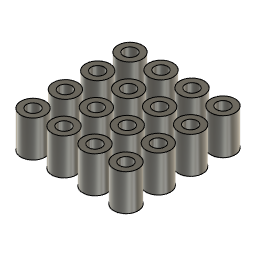
Tall washers v1 (Autodesk Fusion 360 design; units mm, degrees)
Autodesk Fusion 360 part; units mm, degrees
sketch "Sketch1" plane through (0, 0, 0) normal (0, 0, 1) x (1, 0, 0)
  circle A0 centre (0, 0) radius 3
  circle A1 centre (0, 0) radius 1.6
  circle A2 centre (7.6667, 0) radius 1.6
  circle A3 centre (7.6667, 0) radius 3
  circle A4 centre (15.3333, 0) radius 1.6
  circle A5 centre (15.3333, 0) radius 3
  circle A6 centre (23, 0) radius 1.6
  circle A7 centre (23, 0) radius 3
  circle A8 centre (0, -8) radius 1.6
  circle A9 centre (0, -8) radius 3
  circle A10 centre (7.6667, -8) radius 1.6
  circle A11 centre (7.6667, -8) radius 3
  circle A12 centre (15.3333, -8) radius 1.6
  circle A13 centre (15.3333, -8) radius 3
  circle A14 centre (23, -8) radius 1.6
  circle A15 centre (23, -8) radius 3
  circle A16 centre (0, -16) radius 1.6
  circle A17 centre (0, -16) radius 3
  circle A18 centre (7.6667, -16) radius 1.6
  circle A19 centre (7.6667, -16) radius 3
  circle A20 centre (15.3333, -16) radius 1.6
  circle A21 centre (15.3333, -16) radius 3
  circle A22 centre (23, -16) radius 1.6
  circle A23 centre (23, -16) radius 3
  circle A24 centre (0, -24) radius 1.6
  circle A25 centre (0, -24) radius 3
  circle A26 centre (7.6667, -24) radius 1.6
  circle A27 centre (7.6667, -24) radius 3
  circle A28 centre (15.3333, -24) radius 1.6
  circle A29 centre (15.3333, -24) radius 3
  circle A30 centre (23, -24) radius 1.6
  circle A31 centre (23, -24) radius 3
  dimension "d1" = 6
  dimension "d2" = 3.2
  dimension "d5" = 23
  dimension "d6" = -24
  constraint coincident A0.centre A1.centre
  measures "d1" diameter of A0
  measures "d2" diameter of A1
extrude "Extrude1" add sketch "Sketch1" along normal blind 9 makes body 1 at (25.9963, -16.1495, 6) makes body 2 at (18.3296, -8.1495, 6) makes body 3 at (10.6629, -16.1495, 6) makes body 4 at (2.9963, -8.1495, 6) makes body 5 at (2.9963, -16.1495, 6) makes body 6 at (10.6629, -8.1495, 6) makes body 7 at (18.3296, -16.1495, 6) makes body 8 at (25.9963, -8.1495, 6) makes body 9 at (25.9963, -24.1495, 6) makes body 10 at (18.3296, -0.1495, 6) makes body 11 at (10.6629, -24.1495, 6) makes body 12 at (2.9963, -0.1495, 6) makes body 13 at (2.9963, -24.1495, 6) makes body 14 at (10.6629, -0.1495, 6) makes body 15 at (18.3296, -24.1495, 6) makes body 16 at (25.9963, -0.1495, 6)
